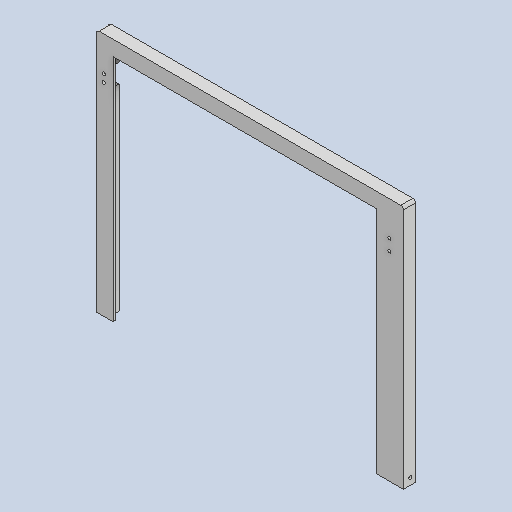
# Autodesk Inventor part: MarcoDerecho
Saved by Autodesk Inventor 2023 (Build 270158000, 158)
## iProperties
Created: 2023-05-12
Part Number: MarcoDerecho
Material: Genérico
Document SubType Name: Modeling
Designer: sergi
Density: 1 g/cm^3
Appearance: Valor por defecto
Author: sergi
Autodesk Inventor part; units mm, degrees
ref_plane "YZ Plane" through (0, 0, 0) normal (1, 0, 0) x (0, 1, 0)
ref_plane "XZ Plane" through (0, 0, 0) normal (0, 1, 0) x (-1, 0, 0)
ref_plane "XY Plane" through (0, 0, 0) normal (0, 0, 1) x (1, 0, 0)
sketch "Boceto1" plane through (0, 0, 0) normal (0, 0, 1) x (1, 0, 0)
  circle A0 centre (100.65, -156.7) radius 1.65 projected
  circle A1 centre (100.65, -148.3) radius 1.65 projected
  circle A2 centre (100.65, 156.7) radius 1.65 projected
  circle A3 centre (100.65, 148.3) radius 1.65 projected
  line L0 (97.75, 145) -> (105.25, 145) projected
  line L1 (105.25, 145) -> (105.25, 160) projected
  line L2 (105.25, 160) -> (97.75, 160) projected
  line L3 (97.75, 160) -> (97.75, 180) projected
  line L4 (97.75, 180) -> (-109, 180) projected
  line L5 (-109, 160) -> (-115.3, 160) projected
  line L6 (-109, -160) -> (-109, -180) projected
  line L7 (-115.3, 146.9) -> (-109, 146.9) projected
  line L8 (-109, -146.9) -> (-115.3, -146.9) projected
  line L9 (-109, 180) -> (-109, 160) projected
  line L10 (-115.3, -160) -> (-109, -160) projected
  line L11 (-109, -180) -> (97.75, -180) projected
  line L12 (97.75, -180) -> (97.75, -160) projected
  line L13 (97.75, -160) -> (105.25, -160) projected
  line L14 (105.25, -160) -> (105.25, -145) projected
  line L15 (105.25, -145) -> (97.75, -145) projected
  line L16 (97.75, -145) -> (97.75, -142) projected
  line L17 (97.75, -142) -> (109, -142) projected
  line L18 (109, -142) -> (109, 142) projected
  line L19 (109, 142) -> (97.75, 142) projected
  line L20 (97.75, 142) -> (97.75, 145) projected
  line L21 (109, 180) -> (97.75, 180)
  line L22 (-109, -160) -> (-109, -180)
  line L23 (-109, -180) -> (-102.7, -180)
  line L24 (-109, -180) -> (109, -180)
  line L25 (109, -180) -> (109, 180)
  line L26 (109, 180) -> (-109, 180)
  line L27 (111, 142) -> (111, 180)
  line L28 (109, 182) -> (97.75, 182)
  line L29 (-109, -182) -> (-102.7, -182)
  line L30 (-111, -182) -> (111, -182)
  line L31 (111, -182) -> (111, 182)
  line L32 (111, 182) -> (-111, 182)
  circle A4 centre (-111.9, -156.3) radius 1.2 projected
  circle A5 centre (-111.9, -150.6) radius 1.2 projected
  circle A6 centre (-111.9, 156.3) radius 1.2 projected
  circle A7 centre (-111.9, 150.6) radius 1.2 projected
  line L33 (-115.3, 160) -> (-115.3, 146.9) projected
  line L34 (-109, 146.9) -> (-109, -146.9) projected
  line L35 (-115.3, -146.9) -> (-115.3, -160) projected
  line L36 (-109, 180) -> (-115.3, 180)
  line L37 (-109, -180) -> (-115.3, -180)
  line L38 (-115.3, 180) -> (109, 180)
  line L39 (109, 180) -> (109, -180)
  line L40 (109, -180) -> (-115.3, -180)
  line L41 (-115.3, -180) -> (-115.3, 180)
  line L42 (-117.3, 180) -> (-117.3, -182)
  line L43 (-117.3, -182) -> (109, -182)
  line L44 (-115.3, 182) -> (111, 182)
  line L45 (111, 182) -> (111, -180)
  line L46 (-117.3, 180) -> (-117.3, 182)
  line L47 (-117.3, 182) -> (-115.3, 182)
  point P0 (0, 0)
  dimension "d1" = 2
  dimension "d3" = 2
  dimension "d20" = 2
  dimension "d21" = 2
  constraints: 48 end point, 6 parallel, 6 perpendicular, 5 horizontal, 2 vertical, 2 other
  measures "d1" distance between parallel lines of L21 L28
  measures "d3" distance between parallel lines of L23 L29
  measures "d20" distance between parallel lines of L41 L42
  measures "d21" distance between parallel lines of L38 L44
extrude "Extrusión1" add sketch "Boceto1" against normal blind 7.5 contours L0 L1 L2 L3 L21 L25 L19 L20 | L25 L24 L12 L13 L14 L15 L16 L17 | L9 L5 L41 L36 | L37 L41 L10 L6 | L7 L34 L8 L41 | L31 L30 L29 L43 L42 L46 L47 L44 L32 L28 L27
sketch "Boceto2" plane through (0, 0, 0) normal (0, 0, 1) x (1, 0, 0)
  line L0 (-117.3, -182) -> (111, -182) projected
  line L1 (111, -182) -> (111, 182) projected
  line L2 (111, 182) -> (-117.3, 182) projected
  line L3 (90.8, 170.8) -> (90.8, -176) projected
  line L4 (90.8, 170.8) -> (90.8, -176) projected
  line L5 (-19.4789, -176) -> (90.8, -176) projected
  line L6 (90.8, -176) -> (-99.7, -176) projected
  line L7 (-99.7, -176) -> (-99.7, 170.8) projected
  line L8 (-99.7, 170.8) -> (90.8, 170.8) projected
  line L9 (-117.3, 182) -> (-117.3, -182) projected
  line L10 (-105.5008, -176) -> (-99.7, -176)
  line L11 (-99.7, 170.8) -> (-105.5008, 170.8)
  line L12 (-109, 160) -> (-109, 180) projected
  line L13 (-109, 170.8) -> (-105, 170.8)
  line L14 (-105, 170.8) -> (-105, -176)
  point P0 (0, 0)
  dimension "d33" = 4
  constraints: 8 end point, 4 point on line, 1 parallel, 1 perpendicular
  measures "d33" distance of L13.start L13.end
extrude "Extrusión2" add sketch "Boceto2" along normal blind 1.5
sketch "Boceto3" plane through (-111, -182, -7.5) normal (0, -1, 0) x (1, 0, 0)
  line L0 (222, 0) -> (-6.3, 0) projected
  line L1 (222, 0) -> (222, 9) projected
  line L2 (-6.3, 9) -> (222, 9) projected
  line L3 (-6.3, 0) -> (-6.3, 9) projected
  point P0 (111, 7.5)
extrude "Extrusión3" add sketch "Boceto3" along normal blind 5.2
sketch "Boceto5" plane through (0, 0, 1.5) normal (0, 0, 1) x (1, 0, 0)
  circle A0 centre (100.65, -156.7) radius 1.65 projected
  circle A1 centre (100.65, -148.3) radius 1.65 projected
  circle A2 centre (100.65, 156.7) radius 1.65 projected
  circle A3 centre (100.65, 148.3) radius 1.65 projected
  line L0 (97.75, 145) -> (105.25, 145) projected
  line L1 (105.25, 145) -> (105.25, 160) projected
  line L2 (105.25, 160) -> (97.75, 160) projected
  line L3 (97.75, 160) -> (97.75, 180) projected
  line L4 (97.75, 180) -> (-109, 180) projected
  line L5 (-109, 160) -> (-115.3, 160) projected
  line L6 (-109, -160) -> (-109, -180) projected
  line L7 (-115.3, 146.9) -> (-109, 146.9) projected
  line L8 (-109, -146.9) -> (-115.3, -146.9) projected
  line L9 (-109, 180) -> (-109, 160) projected
  line L10 (-115.3, -160) -> (-109, -160) projected
  line L11 (-109, -180) -> (97.75, -180) projected
  line L12 (97.75, -180) -> (97.75, -160) projected
  line L13 (97.75, -160) -> (105.25, -160) projected
  line L14 (105.25, -160) -> (105.25, -145) projected
  line L15 (105.25, -145) -> (97.75, -145) projected
  line L16 (97.75, -145) -> (97.75, -142) projected
  line L17 (97.75, -142) -> (109, -142) projected
  line L18 (109, -142) -> (109, 142) projected
  line L19 (109, 142) -> (97.75, 142) projected
  line L20 (97.75, 142) -> (97.75, 145) projected
  circle A4 centre (-111.9, -156.3) radius 1.2 projected
  circle A5 centre (-111.9, -150.6) radius 1.2 projected
  circle A6 centre (-111.9, 156.3) radius 1.2 projected
  circle A7 centre (-111.9, 150.6) radius 1.2 projected
  line L21 (-115.3, 160) -> (-115.3, 146.9) projected
  line L22 (-109, 146.9) -> (-109, -146.9) projected
  line L23 (-115.3, -146.9) -> (-115.3, -160) projected
  point P0 (0, 0)
hole "Agujero1" at (100.65, 148.3, 1.5) at (100.65, 156.7, 1.5) at (100.65, -156.7, 1.5) at (100.65, -148.3, 1.5) at (-111.9, -156.3, 1.5) at (-111.9, -150.6, 1.5) at (-111.9, 150.6, 1.5) at (-111.9, 156.3, 1.5) direction (0, 0, -1) diameter 2.4 end through all
sketch "Boceto6" plane through (0, 0, -7.5) normal (0, 0, -1) x (-1, 0, 0)
  line L0 (117.3, 182) -> (-111, 182) projected
  line L1 (-111, 182) -> (-111, -187.2) projected
  line L2 (117.3, -187.2) -> (-111, -187.2) projected
  line L3 (117.3, 182) -> (117.3, -187.2) projected
  line L4 (-97.75, 160) -> (-97.75, 180) projected
  line L5 (-97.75, 180) -> (109, 180) projected
  line L6 (109, 180) -> (109, 160) projected
  line L7 (109, 160) -> (115.3, 160) projected
  line L8 (115.3, 160) -> (115.3, 146.9) projected
  line L9 (115.3, 146.9) -> (109, 146.9) projected
  line L10 (109, 146.9) -> (109, -146.9) projected
  line L11 (109, -146.9) -> (115.3, -146.9) projected
  line L12 (115.3, -146.9) -> (115.3, -160) projected
  line L13 (115.3, -160) -> (109, -160) projected
  line L14 (109, -160) -> (109, -180) projected
  line L15 (109, -180) -> (-97.75, -180) projected
  line L16 (-97.75, -180) -> (-97.75, -160) projected
  line L17 (-97.75, -160) -> (-105.25, -160) projected
  line L18 (-105.25, -160) -> (-105.25, -145) projected
  line L19 (-105.25, -145) -> (-97.75, -145) projected
  line L20 (-97.75, -145) -> (-97.75, -142) projected
  line L21 (-97.75, -142) -> (-109, -142) projected
  line L22 (-109, -142) -> (-109, 142) projected
  line L23 (-109, 142) -> (-97.75, 142) projected
  line L24 (-97.75, 142) -> (-97.75, 145) projected
  line L25 (-97.75, 145) -> (-105.25, 145) projected
  line L26 (-105.25, 145) -> (-105.25, 160) projected
  line L27 (-105.25, 160) -> (-97.75, 160) projected
  line L28 (117.3, 182) -> (117.3, -187.2) projected
  line L29 (117.3, 182) -> (-111, 182) projected
  line L30 (-111, 182) -> (-111, -187.2) projected
  line L31 (117.3, -187.2) -> (-111, -187.2) projected
  line L32 (109.5, 160.5) -> (109.5, 180.5)
  line L33 (109.5, 180.5) -> (-98.25, 180.5)
  line L34 (-98.25, 180.5) -> (-98.25, 160.5)
  line L35 (-98.25, 160.5) -> (-105.75, 160.5)
  line L36 (-105.75, 160.5) -> (-105.75, 144.5)
  line L37 (-105.75, 144.5) -> (-98.25, 144.5)
  line L38 (-98.25, 144.5) -> (-98.25, 142.5)
  line L39 (-98.25, 142.5) -> (-109.5, 142.5)
  line L40 (-109.5, 142.5) -> (-109.5, -142.5)
  line L41 (-109.5, -142.5) -> (-98.25, -142.5)
  line L42 (-98.25, -142.5) -> (-98.25, -144.5)
  line L43 (-98.25, -144.5) -> (-105.75, -144.5)
  line L44 (-105.75, -144.5) -> (-105.75, -160.5)
  line L45 (-105.75, -160.5) -> (-98.25, -160.5)
  line L46 (-98.25, -160.5) -> (-98.25, -180.5)
  line L47 (-98.25, -180.5) -> (109.5, -180.5)
  line L48 (109.5, -180.5) -> (109.5, -160.5)
  line L49 (109.5, -160.5) -> (115.8, -160.5)
  line L50 (115.8, -160.5) -> (115.8, -146.4)
  line L51 (115.8, -146.4) -> (109.5, -146.4)
  line L52 (109.5, -146.4) -> (109.5, 146.4)
  line L53 (109.5, 146.4) -> (115.8, 146.4)
  line L54 (115.8, 146.4) -> (115.8, 160.5)
  line L55 (115.8, 160.5) -> (109.5, 160.5)
  dimension "d22" = 0.5
  constraints: 48 end point, 23 other
  measures "d22" distance between parallel lines of L6 L32
extrude "Extrusión4" cut sketch "Boceto6" against normal blind 7.5 contours L55 L54 L53 L52 L51 L50 L49 L48 L47 L46 L45 L44 L43 L42 L41 L40 L39 L38 L37 L36 L35 L34 L33 L32
fillet "Empalme1" radius 2 5 edges at (-117.3, 182, 0.75) (-117.3, 182, -3.75) (111, 182, -3) (111, -187.2, -3) (-117.3, -187.2, -3)
sketch "Boceto7" plane through (0, 0, -7.5) normal (0, 0, -1) x (-1, 0, 0)
  arc A0 (117.3, 7) -> (114.3, 10) centre (114.3, 7) ccw projected
  line L0 (114.3, 10) -> (100.3, 10) projected
  arc A1 (100.3, 10) -> (97.3, 7) centre (100.3, 7) ccw projected
  line L1 (97.3, 7) -> (97.3, -7) projected
  arc A2 (97.3, -7) -> (100.3, -10) centre (100.3, -7) ccw projected
  line L2 (100.3, -10) -> (114.3, -10) projected
  arc A3 (114.3, -10) -> (117.3, -7) centre (114.3, -7) ccw projected
  line L3 (117.3, -7) -> (117.3, 7) projected
  circle A4 centre (103.3, -5) radius 1 projected
  circle A5 centre (113.3, 5) radius 1 projected
  circle A6 centre (103.3, 5) radius 1 projected
  circle A7 centre (113.3, -5) radius 1 projected
  circle A8 centre (113.3, 5) radius 1 projected
  point P0 (0, 0)
hole "Agujero2" at (-113.3, 5, -7.5) at (-113.3, -5, -7.5) direction (0, 0, 1) diameter 3 depth 6
split "Dividir4" plane through (0, 0, 0) removes the side toward (0, -1, 0)
sketch "Boceto8" plane through (111, 180, 1.5) normal (1, 0, 0) x (0, 0, -1)
  circle A0 centre (5.1, -175) radius 1.2 projected
  point P0 (1.5, -180)
hole "Agujero3" at (111, 5, -3.6) direction (-1, 0, 0) diameter 2.4 end through all
